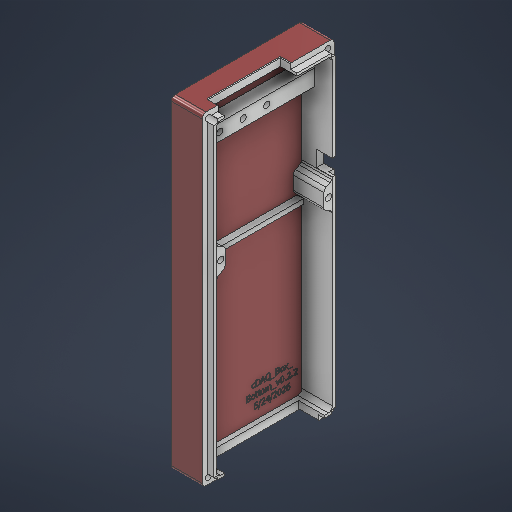
# Autodesk Inventor part: cDAQ_Box_Bottom_v0.2.2ipt
Saved by Autodesk Inventor 2027 (Build 310192000, 192)
## iProperties
Created: 2026-05-08
Part Number: cDAQ_Box_Bottom_v0.2.2ipt
Material: Generic
Document SubType Name: Modeling
Designer: giese
Density: 1 g/cm^3
Appearance: Default
Author: giese
Autodesk Inventor part; units mm, degrees
(part 1 of 2)
ref_plane "YZ Plane" through (0, 0, 0) normal (1, 0, 0) x (0, 1, 0)
ref_plane "XZ Plane" through (0, 0, 0) normal (0, 1, 0) x (-1, 0, 0)
ref_plane "XY Plane" through (0, 0, 0) normal (0, 0, 1) x (1, 0, 0)
sketch "Sketch1" plane through (0, 0, 0) normal (1, 0, 0) x (0, 1, 0)
  line L0 (37.5698, 55.7067) -> (-217.4462, 55.7067)
  line L1 (-217.4462, 55.7067) -> (-217.4462, -48.4333)
  line L2 (-217.4462, -48.4333) -> (37.5698, -48.4333)
  line L3 (37.5698, -48.4333) -> (37.5698, 55.7067)
  point P0 (0, 0)
  dimension "d0" = 104.14
  dimension "d1" = 255.016
  constraints: 8 end point, 2 parallel, 1 horizontal, 1 perpendicular
  measures "d0" distance of L2.end L0.start
  measures "d1" distance of L1.end L2.end
extrude "Extrusion1" add sketch "Sketch1" along normal blind 24.13
sketch "Sketch2" plane through (24.13, 0, 0) normal (1, 0, 0) x (0, 0, -1)
  line L0 (42.0833, 31.2198) -> (-49.3567, 31.2198)
  line L1 (-49.3567, 31.2198) -> (-49.3567, -211.0962)
  line L2 (-49.3567, -211.0962) -> (42.0833, -211.0962)
  line L3 (42.0833, -211.0962) -> (42.0833, 31.2198)
  line L4 (48.4333, 37.5698) -> (-55.7067, 37.5698) projected
  line L5 (-55.7067, 37.5698) -> (-55.7067, -217.4462) projected
  line L6 (-55.7067, -217.4462) -> (48.4333, -217.4462) projected
  line L7 (48.4333, -217.4462) -> (48.4333, 37.5698) projected
  point P0 (0, 0)
  dimension "d4" = 242.316
  dimension "d5" = 91.44
  dimension "d8" = 6.35
  dimension "d21" = 6.35
  dimension "d690" = 6.35
  dimension "d842" = 6.35
  constraints: 8 end point, 2 parallel, 1 horizontal, 1 perpendicular
  measures "d4" distance of L2.end L0.start
  measures "d5" distance of L0.start L0.end
  measures "d8" distance between parallel lines of L0 L4
  measures "d21" distance between parallel lines of L5 L1
  measures "d690" distance between parallel lines of L6 L2
  measures "d842" distance between parallel lines of L7 L3
extrude "Extrusion2" cut sketch "Sketch2" against normal blind 19.05 contours L3 L2 L1 L0
sketch "Sketch3" plane through (0, 0, 0) normal (-1, 0, 0) x (0, 0, 1)
  circle A0 centre (-4.1509, 9.6298) radius 2.4005
  circle A1 centre (14.3479, 9.6298) radius 2.4005
  circle A2 centre (32.8467, 9.6298) radius 2.4005
  line L0 (-48.4333, -217.4462) -> (-48.4333, 37.5698) projected
  line L1 (-48.4333, 37.5698) -> (55.7067, 37.5698) projected
  line L2 (55.7067, 37.5698) -> (55.7067, -217.4462) projected
  line L3 (49.3567, 31.2198) -> (-42.0833, 31.2198) projected
  point P0 (0, 0)
  point P1 (-0.896, -23.7433)
  point P2 (-45.1848, 27.0137)
  dimension "d9" = 18.4988
  dimension "d10" = 4.801
  dimension "d11" = 4.801
  dimension "d12" = 18.4988
  dimension "d13" = 36.9976
  dimension "d18" = 22.86
  dimension "d22" = 4.801
  dimension "d58" = 27.94
  constraints: 3 centre point
  measures "d9" distance of A0.centre A1.centre
  measures "d10" diameter of A1
  measures "d11" diameter of A2
  measures "d12" distance of A1.centre A2.centre
  measures "d13" distance of A0.centre A2.centre
  measures "d18" distance from line of L2 A2.centre
  measures "d22" diameter of A0
  measures "d58" distance from line of L1 A2.centre
extrude "Extrusion3" cut sketch "Sketch3" against normal blind 5.08
sketch "Sketch5" plane through (0, -217.4462, -48.4333) normal (0, 0, -1) x (-1, 0, 0)
  line L0 (-27.2034, 165.862) -> (-16.51, 165.862)
  line L1 (-16.51, 165.862) -> (-16.51, 178.562)
  line L2 (-16.51, 178.562) -> (-27.2034, 178.562)
  line L3 (-27.2034, 178.562) -> (-27.2034, 165.862)
  line L4 (0, 255.016) -> (-24.13, 255.016) projected
  line L5 (0, 0) -> (0, 255.016) projected
  line L6 (-24.13, 0) -> (-24.13, 255.016) projected
  line L7 (0, 0) -> (-24.13, 0) projected
  point P0 (0, 217.4462)
  point P1 (-21.8567, 178.562)
  point P2 (-21.8567, 165.862)
  dimension "d28" = 10.6934
  dimension "d30" = 12.7
  dimension "d31" = 16.51
  dimension "d215" = 3.0734
  dimension "d1133" = 165.862
  constraints: 8 end point, 2 midpoint, 2 parallel, 1 horizontal, 1 perpendicular
  measures "d28" distance between parallel lines of L1 L3
  measures "d30" distance of point (-21.857, 178.562) point (-21.857, 165.862)
  measures "d31" distance between parallel lines of L5 L1
  measures "d215" distance between parallel lines of L6 L3
  measures "d1133" distance between parallel lines of L7 L0
extrude "Extrusion4" cut sketch "Sketch5" against normal blind 24.13 contours L3 L2 L6 L0 | L6 L2 L1 L0
sketch "Sketch6" plane through (0, -217.4462, -48.4333) normal (0, -1, 0) x (1, 0, 0)
  line L0 (24.08, 55.136) -> (16.08, 55.136)
  line L1 (16.08, 45.136) -> (24.08, 45.136)
  line L2 (0, 104.14) -> (0, 0) projected
  line L3 (29.63, 53.1359) -> (29.63, 47.136)
  line L4 (24.08, 55.136) -> (29.63, 53.1359)
  line L5 (29.63, 47.136) -> (24.08, 45.136)
  line L6 (0, 0) -> (24.13, 0) projected
  line L7 (24.13, 97.79) -> (24.13, 6.35) projected
  line L8 (24.13, 41.9134) -> (24.13, 37.4697)
  line L9 (16.08, 55.136) -> (8.636, 55.136)
  line L10 (8.636, 55.136) -> (8.636, 45.136)
  line L11 (8.636, 45.136) -> (21.16, 45.136)
  point P0 (0, 48.4333)
  point P1 (20.08, 55.136)
  point P2 (20.08, 45.136)
  point P3 (16.08, 50.136)
  dimension "d39" = 6
  dimension "d48" = 55.136
  dimension "d221" = 0
  dimension "d223" = 2
  dimension "d224" = 2
  dimension "d225" = 5.5
  dimension "d227" = 5.55
  dimension "d672" = 8.636
  constraints: 18 end point, 2 horizontal, 2 midpoint, 2 parallel, 2 point on line, 1 perpendicular, 1 vertical
  measures "d39" distance of L3.start L3.end
  measures "d48" distance between parallel lines of L6 L0
  measures "d221" horizontal distance of L0.start L1.end
  measures "d223" vertical distance of L3.end L1.end
  measures "d224" vertical distance of L0.start L3.start
  measures "d225" distance between parallel lines of L3 L7
  measures "d227" distance from line of L1.end L3
  measures "d672" distance between parallel lines of L2 L10
extrude "Extrusion5" [suppressed]
sketch "Sketch7" plane through (0, 37.5698, 55.7067) normal (0, 1, 0) x (1, 0, 0)
  line L0 (31.0134, 69.85) -> (16.002, 69.85)
  line L1 (16.002, 69.85) -> (16.002, 12.7)
  line L2 (16.002, 12.7) -> (31.0134, 12.7)
  line L3 (31.0134, 12.7) -> (31.0134, 69.85)
  line L4 (0, 0) -> (24.13, 0) projected
  line L5 (0, 104.14) -> (0, 0) projected
  line L6 (24.13, 104.14) -> (24.13, 0) projected
  point P0 (0, 55.7067)
  point P1 (24.13, 69.85)
  point P2 (24.13, 12.7)
  dimension "d52" = 12.7
  dimension "d55" = 16.002
  dimension "d56" = 15.0114
  dimension "d57" = 6.8834
  dimension "d1195" = 69.85
  constraints: 8 end point, 2 parallel, 1 horizontal, 1 perpendicular
  measures "d52" distance between parallel lines of L4 L2
  measures "d55" distance between parallel lines of L5 L1
  measures "d56" distance between parallel lines of L3 L1
  measures "d57" distance between parallel lines of L6 L3
  measures "d1195" distance between parallel lines of L4 L0
extrude "Extrusion6" cut sketch "Sketch7" against normal blind 7.62
fillet "Fillet1" radius 3.175 4 edges at (12.065, 37.5698, -48.4333) (12.065, 37.5698, 55.7067) (12.065, -217.4462, -48.4333) (12.065, -217.4462, 55.7067)
sketch "Sketch8" plane through (0, 0, 0) normal (-1, 0, 0) x (0, 0, 1)
  line L0 (-5.9225, 6.0992) -> (-2.3919, 6.0992)
  line L1 (-5.9225, 13.1604) -> (-2.3919, 13.1604)
  line L2 (-5.9225, 6.0992) -> (-7.9609, 9.6298)
  line L3 (-5.9225, 13.1604) -> (-7.9609, 9.6298)
  line L4 (-2.3919, 6.0992) -> (-0.3536, 9.6298)
  line L5 (-2.3919, 13.1604) -> (-0.3536, 9.6298)
  circle A0 centre (-4.1509, 9.6298) radius 2.4005 projected
  line L6 (12.5763, 6.0992) -> (16.1069, 6.0992)
  line L7 (12.5763, 13.1604) -> (16.1069, 13.1604)
  line L8 (12.5763, 6.0992) -> (10.5379, 9.6298)
  line L9 (12.5763, 13.1604) -> (10.5379, 9.6298)
  line L10 (16.1069, 6.0992) -> (18.1453, 9.6298)
  line L11 (16.1069, 13.1604) -> (18.1453, 9.6298)
  circle A1 centre (14.3479, 9.6298) radius 2.4005 projected
  line L12 (31.0751, 6.0992) -> (29.0367, 9.6298)
  line L13 (31.0751, 13.1604) -> (29.0367, 9.6298)
  line L14 (31.0751, 6.0992) -> (34.6057, 6.0992)
  line L15 (31.0751, 13.1604) -> (34.6057, 13.1604)
  line L16 (34.6057, 6.0992) -> (36.6441, 9.6298)
  line L17 (34.6057, 13.1604) -> (36.6441, 9.6298)
  circle A2 centre (32.8467, 9.6298) radius 2.4005 projected
  point P0 (-4.1572, 6.0992)
  point P1 (14.3416, 6.0992)
  point P2 (32.8404, 6.0992)
  point P3 (-7.9609, 9.6298)
  point P4 (-0.3536, 9.6298)
  point P5 (18.1453, 9.6298)
  point P6 (10.5379, 9.6298)
  point P7 (36.6441, 9.6298)
  dimension "d60" = 7.0612
  dimension "d61" = 120
  dimension "d62" = 120
  dimension "d63" = 120
  dimension "d64" = 120
  dimension "d65" = 3.5306
  dimension "d66" = 3.5306
  dimension "d67" = 3.5306
  dimension "d68" = 3.5306
  dimension "d69" = 3.5306
  dimension "d70" = 3.5306
  dimension "d71" = 0
  dimension "d72" = 7.6074
  dimension "d73" = 3.81
  dimension "d74" = 0
  dimension "d75" = 7.0612
  dimension "d76" = 120
  dimension "d77" = 120
  dimension "d78" = 120
  dimension "d79" = 120
  dimension "d80" = 3.5306
  dimension "d81" = 3.5306
  dimension "d82" = 3.5306
  dimension "d83" = 3.5306
  dimension "d84" = 3.5306
  dimension "d85" = 3.5306
  dimension "d86" = 0
  dimension "d87" = 7.6074
  dimension "d91" = 0
  dimension "d92" = 3.81
  dimension "d93" = 7.0612
  dimension "d94" = 120
  dimension "d95" = 120
  dimension "d96" = 120
  dimension "d97" = 120
  dimension "d98" = 3.5306
  dimension "d99" = 3.5306
  dimension "d100" = 3.5306
  dimension "d101" = 3.5306
  dimension "d102" = 3.5306
  dimension "d103" = 3.5306
  dimension "d104" = 0
  dimension "d105" = 7.6074
  dimension "d108" = 0
  dimension "d109" = 3.81
  constraints: 36 end point, 6 horizontal, 3 midpoint
  measures "d60" distance from line of point (-4.157, 6.099) L1
  measures "d61" angle of L0 L2
  measures "d62" angle of L1 L3
  measures "d63" angle of L4 L0
  measures "d64" angle of L5 L1
  measures "d65" distance of L0.start L0.end
  measures "d66" distance of L1.start L1.end
  measures "d67" vertical distance of L1.start L3.end
  measures "d68" vertical distance of L0.start L2.end
  measures "d69" vertical distance of L1.end L5.end
  measures "d70" vertical distance of L0.end L4.end
  measures "d71" horizontal distance of L0.start L1.start
  measures "d72" distance of L4.end L2.end
  measures "d73" distance of A0.centre L2.end
  measures "d74" vertical distance of A0.centre L4.end
  measures "d75" distance from line of point (14.342, 6.099) L7
  measures "d76" angle of L6 L8
  measures "d77" angle of L7 L9
  measures "d78" angle of L10 L6
  measures "d79" angle of L11 L7
  measures "d80" distance of L8.start L6.end
  measures "d81" distance of L9.start L7.end
  measures "d82" vertical distance of L9.start L9.end
  measures "d83" vertical distance of L8.start L8.end
  measures "d84" vertical distance of L7.end L11.end
  measures "d85" vertical distance of L6.end L10.end
  measures "d86" horizontal distance of L8.start L9.start
  measures "d87" distance of L10.end L8.end
  measures "d91" vertical distance of A1.centre L8.end
  measures "d92" distance of A1.centre L8.end
  measures "d93" distance from line of point (32.84, 6.099) L15
  measures "d94" angle of L14 L12
  measures "d95" angle of L15 L13
  measures "d96" angle of L16 L14
  measures "d97" angle of L17 L15
  measures "d98" distance of L12.start L16.start
  measures "d99" distance of L15.start L15.end
  measures "d100" vertical distance of L15.start L13.end
  measures "d101" vertical distance of L12.start L12.end
  measures "d102" vertical distance of L15.end L17.end
  measures "d103" vertical distance of L16.start L16.end
  measures "d104" horizontal distance of L12.start L15.start
  measures "d105" distance of L16.end L12.end
  measures "d108" vertical distance of A2.centre L12.end
  measures "d109" distance of A2.centre L12.end
extrude "Extrusion7" cut sketch "Sketch8" against normal blind 4 contours L2 L3 L1 L5 L4 L0 | A0 | L8 L9 L7 L11 L10 L6 | A1 | L12 L13 L15 L17 L16 L14 | A2
sketch "Sketch9" plane through (5.08, 0, 0) normal (1, 0, 0) x (0, 0, -1)
  arc A0 (24.8089, -180.8044) -> (19.3527, -180.8044) centre (22.0808, -178.3302) ccw
  line L0 (45.2583, 37.5698) -> (14.1433, 37.5698) projected
  line L1 (42.0833, 31.2198) -> (42.0833, -38.8842) projected
  arc A1 (20.1758, -185.9502) -> (23.9858, -185.9502) centre (22.0808, -185.9502) ccw
  line L2 (23.9858, -185.9502) -> (23.9858, -182.9374)
  line L3 (20.1758, -185.9502) -> (20.1758, -182.9374)
  arc A2 (24.8089, -180.8044) -> (23.9858, -182.9374) centre (27.1608, -182.9374) ccw
  arc A3 (20.1758, -182.9374) -> (19.3527, -180.8044) centre (17.0008, -182.9374) ccw
  arc A4 (-25.9911, -180.8044) -> (-31.4473, -180.8045) centre (-28.7192, -178.3302) ccw
  arc A5 (-30.6242, -185.9366) -> (-26.8142, -185.9502) centre (-28.7192, -185.9502) ccw
  line L4 (-26.8142, -185.9502) -> (-26.8142, -182.9374)
  line L5 (-30.6242, -185.9366) -> (-30.6242, -182.9374)
  arc A6 (-25.9911, -180.8044) -> (-26.8142, -182.9374) centre (-23.6392, -182.9374) ccw
  arc A7 (-30.6242, -182.9374) -> (-31.4473, -180.8045) centre (-33.7992, -182.9374) ccw
  line L6 (-43.0067, 37.5698) -> (-52.5317, 37.5698) projected
  line L7 (-49.3567, -211.0962) -> (-49.3567, 31.2198) projected
  point P0 (0, 0)
  point P1 (42.0833, -211.0962)
  point P2 (23.9858, -181.4823)
  point P3 (20.1758, -181.4823)
  point P4 (-26.8142, -181.4823)
  point P5 (-30.6242, -181.4823)
  point P6 (-49.3567, -207.2862)
  dimension "d112" = 215.9
  dimension "d114" = 7.366
  dimension "d116" = 3.81
  dimension "d117" = 223.52
  dimension "d118" = 3.175
  dimension "d119" = 7.366
  dimension "d120" = 3.81
  dimension "d121" = 3.175
  dimension "d122" = 215.9
  dimension "d123" = 223.52
  dimension "d125" = 0
  dimension "d128" = 50.8
  dimension "d129" = 20.0025
  dimension "d130" = 0
  constraints: 20 point on circle, 8 centre point, 8 end point, 8 tangent, 4 point on line, 2 equal radius, 2 parallel, 2 vertical
  measures "d112" distance from line of L0 A0.centre
  measures "d114" diameter of A0
  measures "d116" diameter of A1
  measures "d117" distance from line of L0 A1.centre
  measures "d118" radius of A2
  measures "d119" diameter of A4
  measures "d120" diameter of A5
  measures "d121" radius of A6
  measures "d122" distance from line of A4.centre L6
  measures "d123" distance from line of L6 A5.centre
  measures "d125" horizontal distance of A5.centre A4.centre
  measures "d128" distance of A5.centre A1.centre
  measures "d129" distance from line of L1 A0.centre
  measures "d130" horizontal distance of A0.centre A1.centre
extrude "Extrusion8" [suppressed]
sketch "Sketch10" plane through (24.13, 0, 0) normal (1, 0, 0) x (0, 0, -1)
  line L0 (-49.3567, 31.2198) -> (42.0833, 31.2198) projected
  line L1 (-49.3567, 31.2198) -> (42.0833, 31.2198)
  line L2 (42.0833, 33.2264) -> (-46.8167, 33.2264)
  line L3 (-46.8167, 33.2264) -> (-51.3633, 33.2264)
  line L4 (-51.3633, 33.2264) -> (-51.3633, -213.1028)
  line L5 (-51.3633, -213.1028) -> (44.0899, -213.1028)
  line L6 (44.0899, -213.1028) -> (44.0899, 33.2264)
  line L7 (44.0899, 33.2264) -> (41.9392, 33.2264)
  line L8 (42.0833, 31.2198) -> (42.0833, -38.8842) projected
  line L9 (-49.3567, -211.0962) -> (-49.3567, 31.2198) projected
  line L10 (42.0833, -211.0962) -> (-49.3567, -211.0962) projected
  line L11 (45.2583, 37.5698) -> (14.1433, 37.5698) projected
  line L12 (42.0833, 31.2198) -> (42.0833, -211.0962)
  line L13 (42.0833, -211.0962) -> (-49.3567, -211.0962)
  line L14 (-52.5317, -217.4462) -> (45.2583, -217.4462) projected
  line L15 (-49.3567, -211.0962) -> (-49.3567, 31.2198)
  line L16 (-49.3567, 31.2198) -> (42.0833, 31.2198)
  line L17 (-49.3567, 31.2198) -> (42.0833, 31.2198)
  line L18 (42.0833, 31.2198) -> (42.0833, -211.0962)
  line L19 (42.0833, -211.0962) -> (-49.3567, -211.0962)
  line L20 (-49.3567, -211.0962) -> (-49.3567, 31.2198)
  point P0 (-49.3567, -207.2862)
  point P1 (42.0833, -38.8842)
  dimension "d202" = 2.0066
  dimension "d203" = 2.0066
  dimension "d204" = 2.0066
  dimension "d205" = 2.0066
  dimension "d208" = 4.3434
  constraints: 30 end point, 6 perpendicular, 3 collinear, 3 point on line, 2 horizontal, 2 parallel, 1 other
  measures "d202" distance between parallel lines of L0 L2
  measures "d203" distance between parallel lines of L6 L8
  measures "d204" distance between parallel lines of L4 L9
  measures "d205" distance between parallel lines of L5 L10
  measures "d208" distance between parallel lines of L11 L2
extrude "Extrusion9" add sketch "Sketch10" along normal blind 5
fillet "Fillet2" radius 3.175 8 edges at (17.105, 31.2198, -42.0833) (17.105, 31.2198, 49.3567) (17.105, -211.0962, 49.3567) (17.105, -211.0962, -42.0833) (26.63, 33.2264, -44.0899) (26.63, 33.2264, 51.3633) (26.63, -213.1028, -44.0899) (26.63, -213.1028, 51.3633)
sketch "Sketch13" plane through (29.13, 0, 0) normal (1, 0, 0) x (0, 0, -1)
  arc A0 (44.0833, 30.0448) -> (40.9083, 33.2198) centre (40.9083, 30.0448) ccw projected
  arc A1 (-45.6417, 33.2198) -> (-48.8167, 30.0448) centre (-45.6417, 30.0448) ccw projected
  arc A2 (40.9083, -212.0802) -> (44.0833, -208.9052) centre (40.9083, -208.9052) ccw projected
  arc A3 (-48.8167, -208.9052) -> (-45.6417, -212.0802) centre (-45.6417, -208.9052) ccw projected
  line L0 (-43.0067, 37.5698) -> (-52.5317, 37.5698) projected
  line L1 (-55.7067, 34.3948) -> (-55.7067, -214.2712) projected
  line L2 (-52.5317, -217.4462) -> (45.2583, -217.4462) projected
  arc A4 (-48.8167, -208.9052) -> (-45.6417, -212.0802) centre (-45.6417, -208.9052) ccw projected
  circle A5 centre (-50.6267, -212.3662) radius 2.4005
  circle A6 centre (43.3533, -212.3662) radius 2.4005
  line L3 (48.4333, -214.2712) -> (48.4333, 34.3948) projected
  circle A7 centre (43.3533, 32.4898) radius 2.4005
  line L4 (45.2583, 37.5698) -> (14.1433, 37.5698) projected
  circle A8 centre (-50.6267, 32.4898) radius 2.4005
  arc A9 (41.4904, -28.6131) -> (38.3154, -25.4381) centre (38.3154, -28.6131) ccw
  circle A10 centre (38.9083, -64.0302) radius 2.4005
  circle A11 centre (-46.1817, -64.0302) radius 2.4005
  point P0 (0, 0)
  point P1 (-47.8868, 32.2898)
  point P2 (-47.8868, -211.1503)
  point P3 (-47.8868, -211.1503)
  point P4 (45.8404, -24.2631)
  point P5 (42.6654, -21.0881)
  dimension "d178" = 5.08
  dimension "d179" = 5.08
  dimension "d180" = 4.801
  dimension "d181" = 5.08
  dimension "d182" = 5.08
  dimension "d183" = 4.801
  dimension "d184" = 4.801
  dimension "d185" = 5.08
  dimension "d186" = 5.08
  dimension "d187" = 4.801
  dimension "d188" = 5.08
  dimension "d189" = 5.08
  dimension "d326" = 4.801
  dimension "d327" = 9.525
  dimension "d328" = 101.6
  dimension "d329" = 4.801
  dimension "d330" = 9.525
  dimension "d331" = 101.6
  constraints: 7 centre point, 5 point on circle
  measures "d178" distance from line of L1 A5.centre
  measures "d179" distance from line of L2 A5.centre
  measures "d180" diameter of A5
  measures "d181" distance from line of L2 A6.centre
  measures "d182" distance from line of L3 A6.centre
  measures "d183" diameter of A6
  measures "d184" diameter of A7
  measures "d185" distance from line of L3 A7.centre
  measures "d186" distance from line of L4 A7.centre
  measures "d187" diameter of A8
  measures "d188" distance from line of L0 A8.centre
  measures "d189" distance from line of L1 A8.centre
  measures "d326" diameter of A10
  measures "d327" distance from line of L3 A10.centre
  measures "d328" distance from line of A10.centre L4
  measures "d329" diameter of A11
  measures "d330" distance from line of L1 A11.centre
  measures "d331" distance from line of L0 A11.centre
extrude "Extrusion11" cut sketch "Sketch13" against normal blind 25.4
sketch "Sketch14" plane through (5.08, 0, 0) normal (1, 0, 0) x (0, 0, -1)
  line L0 (8.9428, -184.1455) -> (28.1595, -184.1455) construction
  line L1 (28.1595, -184.1455) -> (28.1595, -182.196) construction
  line L2 (28.1595, -182.196) -> (8.9428, -182.196) construction
  line L3 (8.9428, -182.196) -> (8.9428, -184.1455) construction
  spline S0 degree 2 poles (4.046, -188.8916) (3.6903, -188.8916) (3.1012, -188.673) (2.89, -188.4507) knots 0 0 0 1 2 2 2
  spline S1 degree 2 poles (2.89, -188.4507) (2.6788, -188.2321) (2.4454, -187.5578) (2.4454, -187.1058) knots 0 0 0 1 2 2 2
  spline S2 degree 2 poles (2.4454, -187.1058) (2.4454, -186.6538) (2.6862, -185.9943) (2.89, -185.772) knots 0 0 0 1 2 2 2
  spline S3 degree 2 poles (2.89, -185.772) (3.0938, -185.546) (3.6977, -185.3051) (4.046, -185.3051) knots 0 0 0 1 2 2 2
  spline S4 degree 2 poles (4.046, -185.3051) (4.3276, -185.3051) (4.8537, -185.4644) (5.0575, -185.5682) knots 0 0 0 1 2 2 2
  line L4 (5.0575, -185.5682) -> (5.0575, -186.2166)
  line L5 (5.0575, -186.2166) -> (5.0241, -186.2166)
  spline S5 degree 2 poles (5.0241, -186.2166) (4.9611, -186.1647) (4.7685, -186.0313) (4.6314, -185.9609) knots 0 0 0 1 2 2 2
  spline S6 degree 2 poles (4.6314, -185.9609) (4.5091, -185.9016) (4.1831, -185.809) (4.0349, -185.809) knots 0 0 0 1 2 2 2
  spline S7 degree 2 poles (4.0349, -185.809) (3.5866, -185.809) (3.0419, -186.487) (3.0419, -187.1058) knots 0 0 0 1 2 2 2
  spline S8 degree 2 poles (3.0419, -187.1058) (3.0419, -187.7097) (3.568, -188.3877) (4.0349, -188.3877) knots 0 0 0 1 2 2 2
  spline S9 degree 2 poles (4.0349, -188.3877) (4.3165, -188.3877) (4.8277, -188.1543) (5.0241, -187.9727) knots 0 0 0 1 2 2 2
  line L6 (5.0241, -187.9727) -> (5.0575, -187.9727)
  line L7 (5.0575, -187.9727) -> (5.0575, -188.6211)
  spline S10 degree 2 poles (5.0575, -188.6211) (4.9722, -188.6619) (4.7129, -188.7767) (4.6092, -188.8027) knots 0 0 0 1 2 2 2
  spline S11 degree 2 poles (4.6092, -188.8027) (4.461, -188.8471) (4.2275, -188.8916) (4.046, -188.8916) knots 0 0 0 1 2 2 2
  spline S12 degree 2 poles (9.233, -186.5315) (9.233, -187.1576) (8.7254, -188.1654) (8.2994, -188.447) knots 0 0 0 1 2 2 2
  spline S13 degree 2 poles (8.2994, -188.447) (7.9511, -188.6656) (7.236, -188.8138) (6.6803, -188.8138) knots 0 0 0 1 2 2 2
  line L8 (6.6803, -188.8138) -> (5.628, -188.8138)
  line L9 (5.628, -188.8138) -> (5.628, -184.2418)
  line L10 (5.628, -184.2418) -> (6.6691, -184.2418)
  spline S14 degree 2 poles (6.6691, -184.2418) (7.3138, -184.2418) (8.0474, -184.4344) (8.3068, -184.6049) knots 0 0 0 1 2 2 2
  spline S15 degree 2 poles (8.3068, -184.6049) (8.7477, -184.8976) (9.233, -185.8646) (9.233, -186.5315) knots 0 0 0 1 2 2 2
  spline S16 degree 2 poles (8.5995, -186.5241) (8.5995, -185.998) (8.2512, -185.2533) (7.9066, -185.0421) knots 0 0 0 1 2 2 2
  spline S17 degree 2 poles (7.9066, -185.0421) (7.6621, -184.8976) (7.11, -184.7679) (6.6988, -184.7679) knots 0 0 0 1 2 2 2
  line L11 (6.6988, -184.7679) -> (6.2357, -184.7679)
  line L12 (6.2357, -184.7679) -> (6.2357, -188.2877)
  line L13 (6.2357, -188.2877) -> (6.6988, -188.2877)
  spline S18 degree 2 poles (6.6988, -188.2877) (7.1026, -188.2877) (7.714, -188.158) (7.9622, -187.9839) knots 0 0 0 1 2 2 2
  spline S19 degree 2 poles (7.9622, -187.9839) (8.2808, -187.769) (8.5995, -187.0576) (8.5995, -186.5241) knots 0 0 0 1 2 2 2
  line L14 (9.3997, -188.8138) -> (10.941, -184.2418)
  line L15 (10.941, -184.2418) -> (11.6895, -184.2418)
  line L16 (11.6895, -184.2418) -> (13.2307, -188.8138)
  line L17 (13.2307, -188.8138) -> (12.5898, -188.8138)
  line L18 (12.5898, -188.8138) -> (12.1748, -187.5356)
  line L19 (12.1748, -187.5356) -> (10.4297, -187.5356)
  line L20 (10.4297, -187.5356) -> (10.0148, -188.8138)
  line L21 (10.0148, -188.8138) -> (9.3997, -188.8138)
  line L22 (12.0081, -187.0169) -> (11.3004, -184.8642)
  line L23 (11.3004, -184.8642) -> (10.5965, -187.0169)
  line L24 (10.5965, -187.0169) -> (12.0081, -187.0169)
  spline S20 degree 2 poles (17.4619, -189.9327) (17.2952, -189.9735) (16.9321, -190.0179) (16.7505, -190.0179) knots 0 0 0 1 2 2 2
  spline S21 degree 2 poles (16.7505, -190.0179) (16.2355, -190.0179) (15.5945, -189.4436) (15.5649, -188.9101) knots 0 0 0 1 2 2 2
  spline S22 degree 2 poles (15.5649, -188.9101) (15.5242, -188.9101) (15.4538, -188.9101) (15.4241, -188.9101) knots 0 0 0 1 2 2 2
  spline S23 degree 2 poles (15.4241, -188.9101) (14.961, -188.9101) (14.2163, -188.5952) (13.9495, -188.2877) knots 0 0 0 1 2 2 2
  spline S24 degree 2 poles (13.9495, -188.2877) (13.6865, -187.9839) (13.4049, -187.0947) (13.4049, -186.5315) knots 0 0 0 1 2 2 2
  spline S25 degree 2 poles (13.4049, -186.5315) (13.4049, -185.9535) (13.6902, -185.0791) (13.9532, -184.7679) knots 0 0 0 1 2 2 2
  spline S26 degree 2 poles (13.9532, -184.7679) (14.22, -184.4604) (14.9647, -184.1455) (15.4241, -184.1455) knots 0 0 0 1 2 2 2
  spline S27 degree 2 poles (15.4241, -184.1455) (15.891, -184.1455) (16.6394, -184.4715) (16.8987, -184.7679) knots 0 0 0 1 2 2 2
  spline S28 degree 2 poles (16.8987, -184.7679) (17.1581, -185.068) (17.4471, -185.9609) (17.4471, -186.5315) knots 0 0 0 1 2 2 2
  spline S29 degree 2 poles (17.4471, -186.5315) (17.4471, -187.4207) (16.7542, -188.5767) (16.1503, -188.7804) knots 0 0 0 1 2 2 2
  spline S30 degree 2 poles (16.1503, -188.7804) (16.1651, -188.9509) (16.254, -189.225) (16.3244, -189.3029) knots 0 0 0 1 2 2 2
  spline S31 degree 2 poles (16.3244, -189.3029) (16.4097, -189.3992) (16.6431, -189.4881) (16.8506, -189.4881) knots 0 0 0 1 2 2 2
  spline S32 degree 2 poles (16.8506, -189.4881) (16.9728, -189.4881) (17.3063, -189.4103) (17.3804, -189.3807) knots 0 0 0 1 2 2 2
  line L25 (17.3804, -189.3807) -> (17.4619, -189.3807)
  line L26 (17.4619, -189.3807) -> (17.4619, -189.9327)
  spline S33 degree 2 poles (16.8135, -186.5315) (16.8135, -186.0758) (16.6171, -185.3755) (16.4393, -185.1458) knots 0 0 0 1 2 2 2
  spline S34 degree 2 poles (16.4393, -185.1458) (16.2577, -184.9087) (15.7465, -184.6716) (15.4278, -184.6716) knots 0 0 0 1 2 2 2
  spline S35 degree 2 poles (15.4278, -184.6716) (15.0981, -184.6716) (14.6016, -184.9013) (14.4126, -185.1458) knots 0 0 0 1 2 2 2
  spline S36 degree 2 poles (14.4126, -185.1458) (14.2311, -185.3792) (14.0384, -186.0869) (14.0384, -186.5315) knots 0 0 0 1 2 2 2
  spline S37 degree 2 poles (14.0384, -186.5315) (14.0384, -187.4318) (14.7943, -188.3914) (15.4278, -188.3914) knots 0 0 0 1 2 2 2
  spline S38 degree 2 poles (15.4278, -188.3914) (16.0614, -188.3914) (16.8135, -187.4318) (16.8135, -186.5315) knots 0 0 0 1 2 2 2
  line L27 (21.1299, -189.7326) -> (17.6027, -189.7326)
  line L28 (17.6027, -189.7326) -> (17.6027, -189.3362)
  line L29 (17.6027, -189.3362) -> (21.1299, -189.3362)
  line L30 (21.1299, -189.3362) -> (21.1299, -189.7326)
  spline S39 degree 2 poles (24.6459, -187.4096) (24.6459, -187.7504) (24.3866, -188.2729) (24.1717, -188.4433) knots 0 0 0 1 2 2 2
  spline S40 degree 2 poles (24.1717, -188.4433) (23.9123, -188.6434) (23.3232, -188.8138) (22.8564, -188.8138) knots 0 0 0 1 2 2 2
  line L31 (22.8564, -188.8138) -> (21.5448, -188.8138)
  line L32 (21.5448, -188.8138) -> (21.5448, -184.2418)
  line L33 (21.5448, -184.2418) -> (22.7564, -184.2418)
  spline S41 degree 2 poles (22.7564, -184.2418) (23.2454, -184.2418) (23.7345, -184.3048) (23.9568, -184.427) knots 0 0 0 1 2 2 2
  spline S42 degree 2 poles (23.9568, -184.427) (24.205, -184.5567) (24.431, -184.9828) (24.431, -185.2718) knots 0 0 0 1 2 2 2
  spline S43 degree 2 poles (24.431, -185.2718) (24.431, -185.5941) (24.0902, -186.1054) (23.7901, -186.2499) knots 0 0 0 1 2 2 2
  line L34 (23.7901, -186.2499) -> (23.7901, -186.2721)
  spline S44 degree 2 poles (23.7901, -186.2721) (24.1976, -186.3833) (24.6459, -186.9724) (24.6459, -187.4096) knots 0 0 0 1 2 2 2
  spline S45 degree 2 poles (24.0124, -187.4355) (24.0124, -187.1762) (23.8642, -186.8427) (23.6419, -186.7242) knots 0 0 0 1 2 2 2
  spline S46 degree 2 poles (23.6419, -186.7242) (23.4974, -186.6501) (23.1565, -186.6056) (22.8416, -186.6056) knots 0 0 0 1 2 2 2
  line L35 (22.8416, -186.6056) -> (22.1524, -186.6056)
  line L36 (22.1524, -186.6056) -> (22.1524, -188.2951)
  line L37 (22.1524, -188.2951) -> (22.6452, -188.2951)
  spline S47 degree 2 poles (22.6452, -188.2951) (23.0454, -188.2951) (23.5048, -188.221) (23.6826, -188.1024) knots 0 0 0 1 2 2 2
  spline S48 degree 2 poles (23.6826, -188.1024) (23.853, -187.9802) (24.0124, -187.6763) (24.0124, -187.4355) knots 0 0 0 1 2 2 2
  spline S49 degree 2 poles (23.7975, -185.357) (23.7975, -185.194) (23.6863, -184.9494) (23.5641, -184.8791) knots 0 0 0 1 2 2 2
  spline S50 degree 2 poles (23.5641, -184.8791) (23.4159, -184.7975) (23.0565, -184.7605) (22.7341, -184.7605) knots 0 0 0 1 2 2 2
  line L38 (22.7341, -184.7605) -> (22.1524, -184.7605)
  line L39 (22.1524, -184.7605) -> (22.1524, -186.098)
  line L40 (22.1524, -186.098) -> (22.8416, -186.098)
  spline S51 degree 2 poles (22.8416, -186.098) (23.1269, -186.098) (23.3973, -186.0387) (23.5418, -185.9461) knots 0 0 0 1 2 2 2
  spline S52 degree 2 poles (23.5418, -185.9461) (23.6826, -185.8572) (23.7975, -185.5719) (23.7975, -185.357) knots 0 0 0 1 2 2 2
  spline S53 degree 2 poles (28.0249, -187.0984) (28.0249, -187.9653) (27.1913, -188.9101) (26.4947, -188.9101) knots 0 0 0 1 2 2 2
  spline S54 degree 2 poles (26.4947, -188.9101) (25.7797, -188.9101) (24.9609, -187.9357) (24.9609, -187.0984) knots 0 0 0 1 2 2 2
  spline S55 degree 2 poles (24.9609, -187.0984) (24.9609, -186.2388) (25.8056, -185.2866) (26.4947, -185.2866) knots 0 0 0 1 2 2 2
  spline S56 degree 2 poles (26.4947, -185.2866) (27.1913, -185.2866) (28.0249, -186.2351) (28.0249, -187.0984) knots 0 0 0 1 2 2 2
  spline S57 degree 2 poles (27.4284, -187.0984) (27.4284, -186.4315) (26.943, -185.7831) (26.4947, -185.7831) knots 0 0 0 1 2 2 2
  spline S58 degree 2 poles (26.4947, -185.7831) (26.0464, -185.7831) (25.5574, -186.4315) (25.5574, -187.0984) knots 0 0 0 1 2 2 2
  spline S59 degree 2 poles (25.5574, -187.0984) (25.5574, -187.7467) (26.0464, -188.4136) (26.4947, -188.4136) knots 0 0 0 1 2 2 2
  spline S60 degree 2 poles (26.4947, -188.4136) (26.9393, -188.4136) (27.4284, -187.7579) (27.4284, -187.0984) knots 0 0 0 1 2 2 2
  line L41 (31.2816, -188.8138) -> (30.574, -188.8138)
  line L42 (30.574, -188.8138) -> (29.7403, -187.5244)
  line L43 (29.7403, -187.5244) -> (28.8845, -188.8138)
  line L44 (28.8845, -188.8138) -> (28.2287, -188.8138)
  line L45 (28.2287, -188.8138) -> (29.418, -187.1132)
  line L46 (29.418, -187.1132) -> (28.2398, -185.3829)
  line L47 (28.2398, -185.3829) -> (28.9475, -185.3829)
  line L48 (28.9475, -185.3829) -> (29.7774, -186.6612)
  line L49 (29.7774, -186.6612) -> (30.6258, -185.3829)
  line L50 (30.6258, -185.3829) -> (31.2816, -185.3829)
  line L51 (31.2816, -185.3829) -> (30.0997, -187.0761)
  line L52 (30.0997, -187.0761) -> (31.2816, -188.8138)
  line L53 (34.7903, -189.7326) -> (31.2631, -189.7326)
  line L54 (31.2631, -189.7326) -> (31.2631, -189.3362)
  line L55 (31.2631, -189.3362) -> (34.7903, -189.3362)
  line L56 (34.7903, -189.3362) -> (34.7903, -189.7326)
  spline S61 degree 2 poles (1.7748, -194.9373) (1.7748, -195.2781) (1.5155, -195.8005) (1.3006, -195.971) knots 0 0 0 1 2 2 2
  spline S62 degree 2 poles (1.3006, -195.971) (1.0412, -196.171) (0.4521, -196.3415) (-0.0147, -196.3415) knots 0 0 0 1 2 2 2
  line L57 (-0.0147, -196.3415) -> (-1.3263, -196.3415)
  line L58 (-1.3263, -196.3415) -> (-1.3263, -191.7695)
  line L59 (-1.3263, -191.7695) -> (-0.1148, -191.7695)
  spline S63 degree 2 poles (-0.1148, -191.7695) (0.3743, -191.7695) (0.8634, -191.8324) (1.0857, -191.9547) knots 0 0 0 1 2 2 2
  spline S64 degree 2 poles (1.0857, -191.9547) (1.3339, -192.0844) (1.5599, -192.5105) (1.5599, -192.7995) knots 0 0 0 1 2 2 2
  spline S65 degree 2 poles (1.5599, -192.7995) (1.5599, -193.1218) (1.2191, -193.6331) (0.9189, -193.7776) knots 0 0 0 1 2 2 2
  line L60 (0.9189, -193.7776) -> (0.9189, -193.7998)
  spline S66 degree 2 poles (0.9189, -193.7998) (1.3265, -193.911) (1.7748, -194.5001) (1.7748, -194.9373) knots 0 0 0 1 2 2 2
  spline S67 degree 2 poles (1.1412, -194.9632) (1.1412, -194.7038) (0.993, -194.3704) (0.7707, -194.2518) knots 0 0 0 1 2 2 2
  spline S68 degree 2 poles (0.7707, -194.2518) (0.6263, -194.1777) (0.2854, -194.1333) (-0.0295, -194.1333) knots 0 0 0 1 2 2 2
  line L61 (-0.0295, -194.1333) -> (-0.7187, -194.1333)
  line L62 (-0.7187, -194.1333) -> (-0.7187, -195.8228)
  line L63 (-0.7187, -195.8228) -> (-0.2259, -195.8228)
  spline S69 degree 2 poles (-0.2259, -195.8228) (0.1742, -195.8228) (0.6337, -195.7487) (0.8115, -195.6301) knots 0 0 0 1 2 2 2
  spline S70 degree 2 poles (0.8115, -195.6301) (0.9819, -195.5078) (1.1412, -195.204) (1.1412, -194.9632) knots 0 0 0 1 2 2 2
  spline S71 degree 2 poles (0.9264, -192.8847) (0.9264, -192.7217) (0.8152, -192.4771) (0.6929, -192.4067) knots 0 0 0 1 2 2 2
  spline S72 degree 2 poles (0.6929, -192.4067) (0.5447, -192.3252) (0.1854, -192.2882) (-0.137, -192.2882) knots 0 0 0 1 2 2 2
  line L64 (-0.137, -192.2882) -> (-0.7187, -192.2882)
  line L65 (-0.7187, -192.2882) -> (-0.7187, -193.6257)
  line L66 (-0.7187, -193.6257) -> (-0.0295, -193.6257)
  spline S73 degree 2 poles (-0.0295, -193.6257) (0.2557, -193.6257) (0.5262, -193.5664) (0.6707, -193.4738) knots 0 0 0 1 2 2 2
  spline S74 degree 2 poles (0.6707, -193.4738) (0.8115, -193.3849) (0.9264, -193.0996) (0.9264, -192.8847) knots 0 0 0 1 2 2 2
  spline S75 degree 2 poles (5.1538, -194.626) (5.1538, -195.493) (4.3202, -196.4378) (3.6236, -196.4378) knots 0 0 0 1 2 2 2
  spline S76 degree 2 poles (3.6236, -196.4378) (2.9085, -196.4378) (2.0897, -195.4634) (2.0897, -194.626) knots 0 0 0 1 2 2 2
  spline S77 degree 2 poles (2.0897, -194.626) (2.0897, -193.7665) (2.9345, -192.8143) (3.6236, -192.8143) knots 0 0 0 1 2 2 2
  spline S78 degree 2 poles (3.6236, -192.8143) (4.3202, -192.8143) (5.1538, -193.7628) (5.1538, -194.626) knots 0 0 0 1 2 2 2
  spline S79 degree 2 poles (4.5573, -194.626) (4.5573, -193.9591) (4.0719, -193.3108) (3.6236, -193.3108) knots 0 0 0 1 2 2 2
  spline S80 degree 2 poles (3.6236, -193.3108) (3.1753, -193.3108) (2.6862, -193.9591) (2.6862, -194.626) knots 0 0 0 1 2 2 2
  spline S81 degree 2 poles (2.6862, -194.626) (2.6862, -195.2744) (3.1753, -195.9413) (3.6236, -195.9413) knots 0 0 0 1 2 2 2
  spline S82 degree 2 poles (3.6236, -195.9413) (4.0682, -195.9413) (4.5573, -195.2855) (4.5573, -194.626) knots 0 0 0 1 2 2 2
  spline S83 degree 2 poles (6.784, -196.4082) (6.3135, -196.4082) (5.7836, -195.8709) (5.7836, -195.2892) knots 0 0 0 1 2 2 2
  line L67 (5.7836, -195.2892) -> (5.7836, -193.3886)
  line L68 (5.7836, -193.3886) -> (5.3946, -193.3886)
  line L69 (5.3946, -193.3886) -> (5.3946, -192.9106)
  line L70 (5.3946, -192.9106) -> (5.7836, -192.9106)
  line L71 (5.7836, -192.9106) -> (5.7836, -191.9251)
  line L72 (5.7836, -191.9251) -> (6.3616, -191.9251)
  line L73 (6.3616, -191.9251) -> (6.3616, -192.9106)
  line L74 (6.3616, -192.9106) -> (7.425, -192.9106)
  line L75 (7.425, -192.9106) -> (7.425, -193.3886)
  line L76 (7.425, -193.3886) -> (6.3616, -193.3886)
  line L77 (6.3616, -193.3886) -> (6.3616, -195.0225)
  spline S84 degree 2 poles (6.3616, -195.0225) (6.3616, -195.2818) (6.3802, -195.5671) (6.4431, -195.6894) knots 0 0 0 1 2 2 2
  spline S85 degree 2 poles (6.4431, -195.6894) (6.495, -195.7968) (6.7284, -195.9043) (6.9285, -195.9043) knots 0 0 0 1 2 2 2
  spline S86 degree 2 poles (6.9285, -195.9043) (7.0693, -195.9043) (7.3323, -195.8191) (7.3916, -195.7931) knots 0 0 0 1 2 2 2
  line L78 (7.3916, -195.7931) -> (7.425, -195.7931)
  line L79 (7.425, -195.7931) -> (7.425, -196.3118)
  spline S87 degree 2 poles (7.425, -196.3118) (7.2619, -196.3563) (6.9285, -196.4082) (6.784, -196.4082) knots 0 0 0 1 2 2 2
  spline S88 degree 2 poles (8.8885, -196.4082) (8.4179, -196.4082) (7.8881, -195.8709) (7.8881, -195.2892) knots 0 0 0 1 2 2 2
  line L80 (7.8881, -195.2892) -> (7.8881, -193.3886)
  line L81 (7.8881, -193.3886) -> (7.4991, -193.3886)
  line L82 (7.4991, -193.3886) -> (7.4991, -192.9106)
  line L83 (7.4991, -192.9106) -> (7.8881, -192.9106)
  line L84 (7.8881, -192.9106) -> (7.8881, -191.9251)
  line L85 (7.8881, -191.9251) -> (8.4661, -191.9251)
  line L86 (8.4661, -191.9251) -> (8.4661, -192.9106)
  line L87 (8.4661, -192.9106) -> (9.5294, -192.9106)
  line L88 (9.5294, -192.9106) -> (9.5294, -193.3886)
  line L89 (9.5294, -193.3886) -> (8.4661, -193.3886)
  line L90 (8.4661, -193.3886) -> (8.4661, -195.0225)
  spline S89 degree 2 poles (8.4661, -195.0225) (8.4661, -195.2818) (8.4846, -195.5671) (8.5476, -195.6894) knots 0 0 0 1 2 2 2
  spline S90 degree 2 poles (8.5476, -195.6894) (8.5995, -195.7968) (8.8329, -195.9043) (9.033, -195.9043) knots 0 0 0 1 2 2 2
  spline S91 degree 2 poles (9.033, -195.9043) (9.1737, -195.9043) (9.4368, -195.8191) (9.4961, -195.7931) knots 0 0 0 1 2 2 2
  line L91 (9.4961, -195.7931) -> (9.5294, -195.7931)
  line L92 (9.5294, -195.7931) -> (9.5294, -196.3118)
  spline S92 degree 2 poles (9.5294, -196.3118) (9.3664, -196.3563) (9.033, -196.4082) (8.8885, -196.4082) knots 0 0 0 1 2 2 2
  spline S93 degree 2 poles (12.775, -194.626) (12.775, -195.493) (11.9414, -196.4378) (11.2449, -196.4378) knots 0 0 0 1 2 2 2
  spline S94 degree 2 poles (11.2449, -196.4378) (10.5298, -196.4378) (9.711, -195.4634) (9.711, -194.626) knots 0 0 0 1 2 2 2
  spline S95 degree 2 poles (9.711, -194.626) (9.711, -193.7665) (10.5557, -192.8143) (11.2449, -192.8143) knots 0 0 0 1 2 2 2
  spline S96 degree 2 poles (11.2449, -192.8143) (11.9414, -192.8143) (12.775, -193.7628) (12.775, -194.626) knots 0 0 0 1 2 2 2
  spline S97 degree 2 poles (12.1785, -194.626) (12.1785, -193.9591) (11.6932, -193.3108) (11.2449, -193.3108) knots 0 0 0 1 2 2 2
  spline S98 degree 2 poles (11.2449, -193.3108) (10.7965, -193.3108) (10.3075, -193.9591) (10.3075, -194.626) knots 0 0 0 1 2 2 2
  spline S99 degree 2 poles (10.3075, -194.626) (10.3075, -195.2744) (10.7965, -195.9413) (11.2449, -195.9413) knots 0 0 0 1 2 2 2
  spline S100 degree 2 poles (11.2449, -195.9413) (11.6895, -195.9413) (12.1785, -195.2855) (12.1785, -194.626) knots 0 0 0 1 2 2 2
  line L93 (17.2581, -196.3415) -> (17.2581, -194.3556)
  spline S101 degree 2 poles (17.2581, -194.3556) (17.2581, -194.1184) (17.2211, -193.7146) (17.1618, -193.6035) knots 0 0 0 1 2 2 2
  spline S102 degree 2 poles (17.1618, -193.6035) (17.1025, -193.4812) (16.8765, -193.3626) (16.6801, -193.3626) knots 0 0 0 1 2 2 2
  spline S103 degree 2 poles (16.6801, -193.3626) (16.5023, -193.3626) (16.0947, -193.5812) (15.8798, -193.7887) knots 0 0 0 1 2 2 2
  spline S104 degree 2 poles (15.8798, -193.7887) (15.8835, -193.8406) (15.891, -193.9851) (15.891, -194.0814) knots 0 0 0 1 2 2 2
  line L94 (15.891, -194.0814) -> (15.891, -196.3415)
  line L95 (15.891, -196.3415) -> (15.313, -196.3415)
  line L96 (15.313, -196.3415) -> (15.313, -194.3556)
  spline S105 degree 2 poles (15.313, -194.3556) (15.313, -194.1184) (15.2759, -193.7146) (15.2166, -193.6035) knots 0 0 0 1 2 2 2
  spline S106 degree 2 poles (15.2166, -193.6035) (15.1574, -193.4812) (14.9313, -193.3626) (14.735, -193.3626) knots 0 0 0 1 2 2 2
  spline S107 degree 2 poles (14.735, -193.3626) (14.5497, -193.3626) (14.1385, -193.596) (13.9458, -193.7776) knots 0 0 0 1 2 2 2
  line L97 (13.9458, -193.7776) -> (13.9458, -196.3415)
  line L98 (13.9458, -196.3415) -> (13.3678, -196.3415)
  line L99 (13.3678, -196.3415) -> (13.3678, -192.9106)
  line L100 (13.3678, -192.9106) -> (13.9458, -192.9106)
  line L101 (13.9458, -192.9106) -> (13.9458, -193.2885)
  spline S108 degree 2 poles (13.9458, -193.2885) (14.1718, -193.0625) (14.6164, -192.8143) (14.8832, -192.8143) knots 0 0 0 1 2 2 2
  spline S109 degree 2 poles (14.8832, -192.8143) (15.187, -192.8143) (15.6575, -193.0922) (15.7798, -193.4071) knots 0 0 0 1 2 2 2
  spline S110 degree 2 poles (15.7798, -193.4071) (16.0429, -193.1144) (16.5393, -192.8143) (16.8283, -192.8143) knots 0 0 0 1 2 2 2
  spline S111 degree 2 poles (16.8283, -192.8143) (17.0506, -192.8143) (17.4137, -192.9514) (17.5471, -193.107) knots 0 0 0 1 2 2 2
  spline S112 degree 2 poles (17.5471, -193.107) (17.6842, -193.2626) (17.8361, -193.7294) (17.8361, -194.0814) knots 0 0 0 1 2 2 2
  line L102 (17.8361, -194.0814) -> (17.8361, -196.3415)
  line L103 (17.8361, -196.3415) -> (17.2581, -196.3415)
  line L104 (21.7078, -197.2603) -> (18.1807, -197.2603)
  line L105 (18.1807, -197.2603) -> (18.1807, -196.8639)
  line L106 (18.1807, -196.8639) -> (21.7078, -196.8639)
  line L107 (21.7078, -196.8639) -> (21.7078, -197.2603)
  line L108 (24.7719, -192.9106) -> (23.4788, -196.3415)
  line L109 (23.4788, -196.3415) -> (22.9601, -196.3415)
  line L110 (22.9601, -196.3415) -> (21.6782, -192.9106)
  line L111 (21.6782, -192.9106) -> (22.3043, -192.9106)
  line L112 (22.3043, -192.9106) -> (23.2417, -195.5523)
  line L113 (23.2417, -195.5523) -> (24.1717, -192.9106)
  line L114 (24.1717, -192.9106) -> (24.7719, -192.9106)
  spline S113 degree 2 poles (27.9693, -194.0555) (27.9693, -195.2855) (27.2543, -196.4378) (26.5096, -196.4378) knots 0 0 0 1 2 2 2
  spline S114 degree 2 poles (26.5096, -196.4378) (25.7537, -196.4378) (25.0461, -195.2633) (25.0461, -194.0592) knots 0 0 0 1 2 2 2
  spline S115 degree 2 poles (25.0461, -194.0592) (25.0461, -192.8217) (25.7611, -191.6768) (26.5096, -191.6768) knots 0 0 0 1 2 2 2
  spline S116 degree 2 poles (26.5096, -191.6768) (27.2617, -191.6768) (27.9693, -192.8624) (27.9693, -194.0555) knots 0 0 0 1 2 2 2
  spline S117 degree 2 poles (27.1839, -195.4486) (27.2728, -195.2225) (27.3469, -194.526) (27.3469, -194.0555) knots 0 0 0 1 2 2 2
  spline S118 degree 2 poles (27.3469, -194.0555) (27.3469, -193.5849) (27.2728, -192.8921) (27.1802, -192.6587) knots 0 0 0 1 2 2 2
  spline S119 degree 2 poles (27.1802, -192.6587) (27.0875, -192.4253) (26.7652, -192.1844) (26.5096, -192.1844) knots 0 0 0 1 2 2 2
  spline S120 degree 2 poles (26.5096, -192.1844) (26.2539, -192.1844) (25.9242, -192.4253) (25.8278, -192.6661) knots 0 0 0 1 2 2 2
  spline S121 degree 2 poles (25.8278, -192.6661) (25.7352, -192.8995) (25.6685, -193.6109) (25.6685, -194.0592) knots 0 0 0 1 2 2 2
  spline S122 degree 2 poles (25.6685, -194.0592) (25.6685, -194.5408) (25.7278, -195.1855) (25.8241, -195.4374) knots 0 0 0 1 2 2 2
  spline S123 degree 2 poles (25.8241, -195.4374) (25.913, -195.6746) (26.2428, -195.9302) (26.5096, -195.9302) knots 0 0 0 1 2 2 2
  spline S124 degree 2 poles (26.5096, -195.9302) (26.7615, -195.9302) (27.0912, -195.6894) (27.1839, -195.4486) knots 0 0 0 1 2 2 2
  line L115 (29.5366, -196.3415) -> (28.803, -196.3415)
  line L116 (28.803, -196.3415) -> (28.803, -195.4671)
  line L117 (28.803, -195.4671) -> (29.5366, -195.4671)
  line L118 (29.5366, -195.4671) -> (29.5366, -196.3415)
  line L119 (33.2786, -196.3415) -> (30.4591, -196.3415)
  line L120 (30.4591, -196.3415) -> (30.4591, -195.6931)
  spline S125 degree 2 poles (30.4591, -195.6931) (30.7629, -195.4078) (31.3039, -194.878) (31.5632, -194.5927) knots 0 0 0 1 2 2 2
  spline S126 degree 2 poles (31.5632, -194.5927) (32.0856, -194.0184) (32.4672, -193.3293) (32.4672, -192.9625) knots 0 0 0 1 2 2 2
  spline S127 degree 2 poles (32.4672, -192.9625) (32.4672, -192.7698) (32.3487, -192.4808) (32.2412, -192.3882) knots 0 0 0 1 2 2 2
  spline S128 degree 2 poles (32.2412, -192.3882) (32.1338, -192.2956) (31.8522, -192.203) (31.6818, -192.203) knots 0 0 0 1 2 2 2
  spline S129 degree 2 poles (31.6818, -192.203) (31.5187, -192.203) (31.1853, -192.2845) (31.0334, -192.3474) knots 0 0 0 1 2 2 2
  spline S130 degree 2 poles (31.0334, -192.3474) (30.9037, -192.3993) (30.6629, -192.5475) (30.5888, -192.5994) knots 0 0 0 1 2 2 2
  line L121 (30.5888, -192.5994) -> (30.5554, -192.5994)
  line L122 (30.5554, -192.5994) -> (30.5554, -191.9473)
  spline S131 degree 2 poles (30.5554, -191.9473) (30.7444, -191.8547) (31.4224, -191.6731) (31.7262, -191.6731) knots 0 0 0 1 2 2 2
  spline S132 degree 2 poles (31.7262, -191.6731) (32.3672, -191.6731) (33.0897, -192.3512) (33.0897, -192.9291) knots 0 0 0 1 2 2 2
  spline S133 degree 2 poles (33.0897, -192.9291) (33.0897, -193.1996) (32.9637, -193.6516) (32.8526, -193.8443) knots 0 0 0 1 2 2 2
  spline S134 degree 2 poles (32.8526, -193.8443) (32.7414, -194.0443) (32.4191, -194.4371) (32.2412, -194.626) knots 0 0 0 1 2 2 2
  spline S135 degree 2 poles (32.2412, -194.626) (31.9522, -194.941) (31.2446, -195.6153) (31.0334, -195.8116) knots 0 0 0 1 2 2 2
  line L123 (31.0334, -195.8116) -> (33.2786, -195.8116)
  line L124 (33.2786, -195.8116) -> (33.2786, -196.3415)
  line L125 (34.8718, -196.3415) -> (34.1382, -196.3415)
  line L126 (34.1382, -196.3415) -> (34.1382, -195.4671)
  line L127 (34.1382, -195.4671) -> (34.8718, -195.4671)
  line L128 (34.8718, -195.4671) -> (34.8718, -196.3415)
  line L129 (38.6139, -196.3415) -> (35.7943, -196.3415)
  line L130 (35.7943, -196.3415) -> (35.7943, -195.6931)
  spline S136 degree 2 poles (35.7943, -195.6931) (36.0982, -195.4078) (36.6391, -194.878) (36.8984, -194.5927) knots 0 0 0 1 2 2 2
  spline S137 degree 2 poles (36.8984, -194.5927) (37.4208, -194.0184) (37.8025, -193.3293) (37.8025, -192.9625) knots 0 0 0 1 2 2 2
  spline S138 degree 2 poles (37.8025, -192.9625) (37.8025, -192.7698) (37.6839, -192.4808) (37.5765, -192.3882) knots 0 0 0 1 2 2 2
  spline S139 degree 2 poles (37.5765, -192.3882) (37.469, -192.2956) (37.1874, -192.203) (37.017, -192.203) knots 0 0 0 1 2 2 2
  spline S140 degree 2 poles (37.017, -192.203) (36.854, -192.203) (36.5205, -192.2845) (36.3686, -192.3474) knots 0 0 0 1 2 2 2
  spline S141 degree 2 poles (36.3686, -192.3474) (36.2389, -192.3993) (35.9981, -192.5475) (35.924, -192.5994) knots 0 0 0 1 2 2 2
  line L131 (35.924, -192.5994) -> (35.8907, -192.5994)
  line L132 (35.8907, -192.5994) -> (35.8907, -191.9473)
  spline S142 degree 2 poles (35.8907, -191.9473) (36.0796, -191.8547) (36.7576, -191.6731) (37.0615, -191.6731) knots 0 0 0 1 2 2 2
  spline S143 degree 2 poles (37.0615, -191.6731) (37.7024, -191.6731) (38.4249, -192.3512) (38.4249, -192.9291) knots 0 0 0 1 2 2 2
  spline S144 degree 2 poles (38.4249, -192.9291) (38.4249, -193.1996) (38.2989, -193.6516) (38.1878, -193.8443) knots 0 0 0 1 2 2 2
  spline S145 degree 2 poles (38.1878, -193.8443) (38.0766, -194.0443) (37.7543, -194.4371) (37.5765, -194.626) knots 0 0 0 1 2 2 2
  spline S146 degree 2 poles (37.5765, -194.626) (37.2875, -194.941) (36.5798, -195.6153) (36.3686, -195.8116) knots 0 0 0 1 2 2 2
  line L133 (36.3686, -195.8116) -> (38.6139, -195.8116)
  line L134 (38.6139, -195.8116) -> (38.6139, -196.3415)
  spline S147 degree 2 poles (7.362, -202.3871) (7.362, -202.7391) (7.1286, -203.3356) (6.9322, -203.5357) knots 0 0 0 1 2 2 2
  spline S148 degree 2 poles (6.9322, -203.5357) (6.7284, -203.7469) (6.2171, -203.9655) (5.9096, -203.9655) knots 0 0 0 1 2 2 2
  spline S149 degree 2 poles (5.9096, -203.9655) (5.6021, -203.9655) (5.0945, -203.758) (4.9018, -203.5505) knots 0 0 0 1 2 2 2
  spline S150 degree 2 poles (4.9018, -203.5505) (4.6647, -203.3023) (4.398, -202.4686) (4.398, -201.861) knots 0 0 0 1 2 2 2
  spline S151 degree 2 poles (4.398, -201.861) (4.398, -201.2645) (4.6425, -200.3049) (4.8981, -199.9492) knots 0 0 0 1 2 2 2
  spline S152 degree 2 poles (4.8981, -199.9492) (5.1464, -199.601) (5.9318, -199.2119) (6.4468, -199.2119) knots 0 0 0 1 2 2 2
  spline S153 degree 2 poles (6.4468, -199.2119) (6.5988, -199.2119) (6.8655, -199.2416) (6.9655, -199.2749) knots 0 0 0 1 2 2 2
  line L135 (6.9655, -199.2749) -> (6.9655, -199.864)
  line L136 (6.9655, -199.864) -> (6.9396, -199.864)
  spline S154 degree 2 poles (6.9396, -199.864) (6.8544, -199.8196) (6.5432, -199.7417) (6.3653, -199.7417) knots 0 0 0 1 2 2 2
  spline S155 degree 2 poles (6.3653, -199.7417) (5.7948, -199.7417) (5.0945, -200.5124) (5.0278, -201.2682) knots 0 0 0 1 2 2 2
  spline S156 degree 2 poles (5.0278, -201.2682) (5.2464, -201.1163) (5.7058, -200.9496) (5.98, -200.9496) knots 0 0 0 1 2 2 2
  spline S157 degree 2 poles (5.98, -200.9496) (6.2468, -200.9496) (6.6469, -201.057) (6.8655, -201.22) knots 0 0 0 1 2 2 2
  spline S158 degree 2 poles (6.8655, -201.22) (7.1175, -201.409) (7.362, -201.9944) (7.362, -202.3871) knots 0 0 0 1 2 2 2
  spline S159 degree 2 poles (6.7395, -202.4131) (6.7395, -202.1315) (6.5913, -201.7499) (6.4283, -201.6165) knots 0 0 0 1 2 2 2
  spline S160 degree 2 poles (6.4283, -201.6165) (6.3061, -201.5202) (6.0022, -201.4572) (5.8429, -201.4572) knots 0 0 0 1 2 2 2
  spline S161 degree 2 poles (5.8429, -201.4572) (5.628, -201.4572) (5.2242, -201.5868) (5.0278, -201.7091) knots 0 0 0 1 2 2 2
  spline S162 degree 2 poles (5.0278, -201.7091) (5.0241, -201.7758) (5.0167, -201.9018) (5.0167, -201.9981) knots 0 0 0 1 2 2 2
  spline S163 degree 2 poles (5.0167, -201.9981) (5.0167, -202.4723) (5.202, -203.054) (5.3427, -203.2059) knots 0 0 0 1 2 2 2
  spline S164 degree 2 poles (5.3427, -203.2059) (5.4724, -203.3504) (5.754, -203.4653) (5.9133, -203.4653) knots 0 0 0 1 2 2 2
  spline S165 degree 2 poles (5.9133, -203.4653) (6.2838, -203.4653) (6.7395, -202.9392) (6.7395, -202.4131) knots 0 0 0 1 2 2 2
  line L137 (9.8036, -199.0934) -> (8.0141, -204.8621)
  line L138 (8.0141, -204.8621) -> (7.4954, -204.8621)
  line L139 (7.4954, -204.8621) -> (9.2775, -199.0934)
  line L140 (9.2775, -199.0934) -> (9.8036, -199.0934)
  line L141 (13.127, -203.8691) -> (10.3075, -203.8691)
  line L142 (10.3075, -203.8691) -> (10.3075, -203.2208)
  spline S166 degree 2 poles (10.3075, -203.2208) (10.6113, -202.9355) (11.1522, -202.4057) (11.4116, -202.1204) knots 0 0 0 1 2 2 2
  spline S167 degree 2 poles (11.4116, -202.1204) (11.934, -201.5461) (12.3156, -200.857) (12.3156, -200.4902) knots 0 0 0 1 2 2 2
  spline S168 degree 2 poles (12.3156, -200.4902) (12.3156, -200.2975) (12.197, -200.0085) (12.0896, -199.9159) knots 0 0 0 1 2 2 2
  spline S169 degree 2 poles (12.0896, -199.9159) (11.9822, -199.8233) (11.7006, -199.7306) (11.5301, -199.7306) knots 0 0 0 1 2 2 2
  spline S170 degree 2 poles (11.5301, -199.7306) (11.3671, -199.7306) (11.0337, -199.8121) (10.8818, -199.8751) knots 0 0 0 1 2 2 2